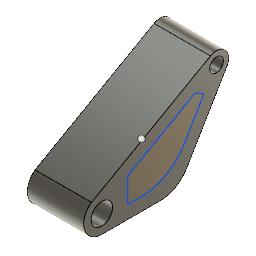
6.7 split face & body (Autodesk Fusion 360 design; units mm, degrees)
Autodesk Fusion 360 part; units mm, degrees
sketch "Sketch1" plane through (0, 0, 0) normal (1, 0, 0) x (0, 1, 0)
  circle A0 centre (0, 0) radius 9.332
  line L0 (-0.293, -15.7817) -> (50.7077, -15.7817)
  line L1 (74.0537, -2.44) -> (108.9435, 56.7771)
  line L2 (-8.9747, 12.9847) -> (94.4391, 71.534)
  arc A1 (50.7077, -15.7817) -> (74.0537, -2.44) centre (50.7077, 11.3152) ccw
  arc A2 (-6.5163, 14.3766) -> (0.293, -15.7817) centre (0, 0) ccw
  arc A3 (108.9435, 56.7771) -> (94.4391, 71.534) centre (99.7158, 62.2139) ccw
  circle A4 centre (99.7158, 62.2139) radius 6.0013
  dimension "d1" = 27.0969
  dimension "d3" = 15.7844
  dimension "d4" = 18.6641
  dimension "d5" = 12.0025
  dimension "d6" = 10.7102
  dimension "d7" = 59.494
  dimension "d8" = 29.517
  dimension "d12" = 77.9956
  dimension "d13" = 99.7158
  dimension "d16" = 118.8379
  constraint coincident A0.centre A2.centre
  constraint concentric A0 A2
  constraint coincident L0.start A2
  constraint horizontal L0
  constraint tangent L2 A3
  constraint tangent L1 A3
  constraint tangent L0 A1
  constraint tangent L1 A1
  constraint coincident L2.start A2
  constraint coincident L0 A2.end
  constraint coincident L2 A2.start
  constraint concentric A3 A4
  measures "d1" radius of A1
  measures "d3" radius of A2
  measures "d4" diameter of A0
  measures "d5" diameter of A4
  measures "d6" radius of A3
  measures "d7" angle of L0 L1
  measures "d8" angle of L0 L2
  measures "d12" distance of L0 A3.centre
  measures "d13" horizontal distance of A0.centre A3.centre
  measures "d16" distance of L2.end L2.start
sketch "Sketch3" plane through (0, 0, 0) normal (1, 0, 0) x (0, 1, 0)
  line L0 (81.0105, 50.2421) -> (22.4827, 17.1057)
  line L1 (22.4827, 17.1057) -> (22.4827, -4.1678)
  line L2 (22.4827, -4.1678) -> (34.4677, -4.1678)
  line L3 (71.7994, 17.1664) -> (88.731, 45.9038)
  line L4 (88.731, 45.9038) -> (81.0105, 50.2421)
  arc A0 (34.4677, -4.1678) -> (71.7994, 17.1664) centre (34.4677, 39.1617) ccw
  dimension "d17" = 43.3295
  constraint vertical L1
  constraint perpendicular L1 L2
  constraint tangent L2 A0
  constraint tangent L3 A0
  measures "d17" radius of A0
extrude "Extrude1" add sketch "Sketch1" against normal blind 49.171 contours L0 L1 L2 A1 A2 A3
